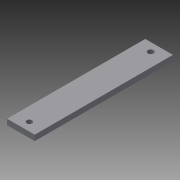
# Autodesk Inventor part: Frame
Saved by Autodesk Inventor 2015 (Build 190159000, 159)
## iProperties
Created: 2015-01-27
Part Number: Frame
Material: Generic
Document SubType Name: Modeling
Designer: chapale16
Density: 1 g/cm^3
Appearance: Default
Author: chapale16
Autodesk Inventor part; units mm, degrees
ref_plane "YZ Plane" through (0, 0, 0) normal (1, 0, 0) x (0, 1, 0)
ref_plane "XZ Plane" through (0, 0, 0) normal (0, 1, 0) x (-1, 0, 0)
ref_plane "XY Plane" through (0, 0, 0) normal (0, 0, 1) x (1, 0, 0)
sketch "Sketch1" plane through (0, 0, 0) normal (0, 1, 0) x (-1, 0, 0)
  line L0 (0, 0) -> (-127, 0)
  line L1 (-127, 0) -> (-127, -635)
  line L2 (-127, -635) -> (0, -635)
  line L3 (0, -635) -> (0, 0)
  circle A0 centre (-63.5, -38.9382) radius 12.5273
  circle A1 centre (-63.5, -596.0618) radius 13.2642
  dimension "d0" = 127
  dimension "d1" = 635
  dimension "d2" = 38.9382
  dimension "d3" = 38.9382
  constraints: 8 end point, 2 centre point, 2 parallel, 1 horizontal, 1 perpendicular
  measures "d0" distance of L2.end L1.end
  measures "d1" distance of L1.end L0.end
  measures "d2" distance from line of L0 A0.centre
  measures "d3" distance from line of L2 A1.centre
extrude "Extrusion1" add sketch "Sketch1" along normal blind 25.4
body "Solid1"
